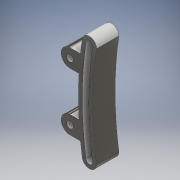
# Autodesk Inventor part: reverse gear gear link
Saved by Autodesk Inventor 2017 (Build 210142000, 142)
## iProperties
Created: 2018-11-06
Part Number: reverse gear gear link
Material: Generic
Document SubType Name: Modeling
Designer: User
Density: 1 g/cm^3
Appearance: Default
Author: User
Autodesk Inventor part; units mm, degrees
ref_plane "YZ Plane" through (0, 0, 0) normal (1, 0, 0) x (0, 1, 0)
ref_plane "XZ Plane" through (0, 0, 0) normal (0, 1, 0) x (-1, 0, 0)
ref_plane "XY Plane" through (0, 0, 0) normal (0, 0, 1) x (1, 0, 0)
sketch "Sketch1" plane through (0, 0, 0) normal (0, 1, 0) x (-1, 0, 0)
  arc A0 (0, -45) -> (0.2133, -43.5152) centre (-151.3365, -22.5) ccw
  circle A1 centre (0, 0) radius 1.5
  circle A2 centre (0, -45) radius 1.5
  arc A3 (-3.1094, -44.0545) -> (3.25, -45) centre (0, -45) ccw
  arc A4 (3.25, 0) -> (-3.1094, -0.9455) centre (0, 0) ccw
  arc A5 (3.25, -45) -> (3.25, 0) centre (-151.3365, -22.5) ccw
  arc A6 (-3.25, -45) -> (-3.25, 0) centre (-151.3365, -22.5) ccw
  arc A7 (-1.5, -45) -> (-1.5, 0) centre (-151.3365, -22.5) ccw
  arc A8 (1.5, -45) -> (1.5, 0) centre (-151.3365, -22.5) ccw
  circle A9 centre (8.6635, -35.4615) radius 1.5
  circle A10 centre (8.6635, -9.5385) radius 1.5
  circle A11 centre (8.6635, -9.5385) radius 4
  circle A12 centre (8.6635, -35.4615) radius 4
  line L0 (8.6635, -5.5385) -> (3.9553, -5.5385)
  line L1 (8.6635, -13.5385) -> (4.6216, -13.5385)
  line L2 (8.6635, -31.4615) -> (4.6216, -31.4615)
  line L3 (8.6635, -39.4615) -> (3.9553, -39.4615)
  dimension "d0" = 3
  dimension "d1" = 6.5
  dimension "d3" = 8
  dimension "d4" = 156.2154
  dimension "d5" = 154.4838
  dimension "d6" = 153
  dimension "d7" = 151.5165
  dimension "d8" = 149.7861
  dimension "d9" = 17.923
  dimension "d10" = 13.5385
  dimension "d11" = 13.5385
  dimension "d12" = 31.4615
  dimension "d13" = 13.5385
  dimension "d14" = 31.4615
  dimension "d15" = 10.2825
  dimension "d16" = 32.6325
  dimension "d17" = 14.3056
  constraints: 31 point on circle, 13 centre point, 8 end point, 6 coincident, 5 equal radius, 4 concentric, 4 tangent, 3 parallel, 1 horizontal
  measures "d0" diameter of A1
  measures "d1" diameter of A4
  measures "d3" diameter of A11
  measures "d4" radius of A5
  measures "d5" radius of A8
  measures "d6" radius of A0
  measures "d7" radius of A7
  measures "d8" radius of A6
  measures "d9" distance between parallel lines of L1 L2
  measures "d10" distance from line of point (0, 0) L1
  measures "d11" distance from line of A4.start L1
  measures "d12" distance from line of A3.end L1
  measures "d13" distance from line of A1.end L1
  measures "d14" distance from line of A8.start L1
  measures "d15" distance of point (0, 0) L0.start
  measures "d16" distance of point (0, 0) L2.start
  measures "d17" distance of point (0, 0) L1.end
extrude "Extrusion2" add sketch "Sketch1" along normal blind 10 contours A6 A4 A5 A3 | A5 L2 A12 L3 | A12 | L0 A11 L1 A5 | A11
sketch "Sketch2" plane through (0, 10, 0) normal (0, 1, 0) x (1, 0, 0)
  arc A0 (-1.5, 45) -> (-1.5, 0) centre (151.3365, 22.5) ccw projected
  arc A1 (1.4351, 44.5636) -> (-1.5, 45) centre (0, 45) ccw projected
  arc A2 (1.4351, 44.5636) -> (1.4351, 0.4364) centre (151.3365, 22.5) ccw projected
  arc A3 (-1.5, 0) -> (1.4351, 0.4364) centre (0, 0) ccw projected
  circle A4 centre (-8.6635, 35.4615) radius 1.5 projected
  circle A5 centre (-8.6635, 9.5385) radius 1.5 projected
  line L0 (-4.6216, 13.5385) -> (-8.6635, 13.5385) projected
  arc A6 (-8.6635, 13.5385) -> (-8.6635, 5.5385) centre (-8.6635, 9.5385) ccw projected
  line L1 (-8.6635, 5.5385) -> (-3.9553, 5.5385) projected
  arc A7 (-3.9553, 5.5385) -> (-3.25, 0) centre (151.3365, 22.5) ccw projected
  arc A8 (-3.25, 0) -> (3.25, 0) centre (0, 0) ccw projected
  arc A9 (3.25, 45) -> (3.25, 0) centre (151.3365, 22.5) ccw projected
  arc A10 (3.25, 45) -> (-3.25, 45) centre (0, 45) ccw projected
  arc A11 (-3.25, 45) -> (-3.9553, 39.4615) centre (151.3365, 22.5) ccw projected
  line L2 (-3.9553, 39.4615) -> (-8.6635, 39.4615) projected
  arc A12 (-8.6635, 39.4615) -> (-8.6635, 31.4615) centre (-8.6635, 35.4615) ccw projected
  line L3 (-8.6635, 31.4615) -> (-4.6216, 31.4615) projected
  arc A13 (-4.6216, 31.4615) -> (-4.6216, 13.5385) centre (151.3365, 22.5) ccw projected
  circle A14 centre (-8.6635, 9.5385) radius 1.5 projected
  circle A15 centre (-8.6635, 9.5385) radius 3.25
  circle A16 centre (-8.6635, 35.4615) radius 3.25
  dimension "d22" = 6.5
  dimension "d23" = 6.5
  constraints: 2 centre point, 2 coincident
  measures "d22" diameter of A15
  measures "d23" diameter of A16
extrude "Extrusion3" cut sketch "Sketch2" against normal blind 1.75 contours A15 | A16
chamfer "Chamfer1" distance 1.75 angle 45 1 edges at (-7.1635, 8.25, -9.5385)
chamfer "Chamfer2" distance 1.75 angle 45 1 edges at (-7.1635, 8.25, -35.4615)
body "Solid2"
